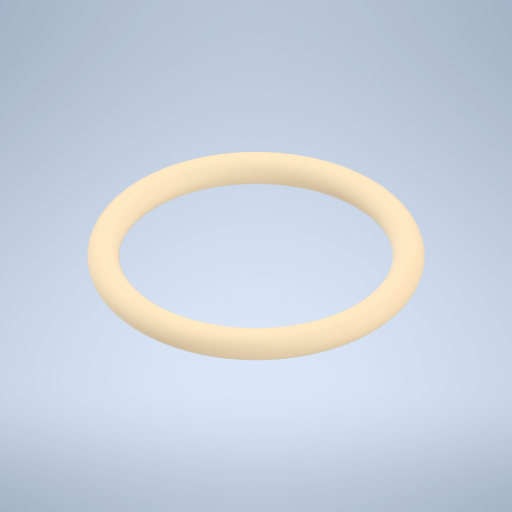
# Autodesk Inventor part: dummy_ling_string
Saved by Autodesk Inventor 2024.3 (Build 283343000, 343)
## iProperties
Created: 2024-09-12
Part Number: dummy_ling_string
Material: Generic
Document SubType Name: Modeling
Designer: gihyeok2
Density: 1 g/cm^3
Appearance: Default
Author: gihyeok2
Autodesk Inventor part; units mm, degrees
ref_plane "YZ Plane" through (0, 0, 0) normal (1, 0, 0) x (0, 1, 0)
ref_plane "XZ Plane" through (0, 0, 0) normal (0, 1, 0) x (-1, 0, 0)
ref_plane "XY Plane" through (0, 0, 0) normal (0, 0, 1) x (1, 0, 0)
sketch "Sketch3" plane through (0, 0, 0) normal (1, 0, 0) x (0, 1, 0)
  circle A0 centre (0, -2.35) radius 0.25
  line L0 (0, -2.35) -> (0, 0) construction
  line L1 (0, 0) -> (6.6454, 0) construction
  dimension "d3" = 0.5
  dimension "d4" = 2.35
  constraints: 4 end point, 1 centre point, 1 horizontal, 1 vertical
  measures "d3" diameter of A0
  measures "d4" distance of L0.start L0.end
revolve "Revolution1" add sketch "Sketch3" angle 360 about axis through (0, 0, 0) along (0, 1, 0)
body "Solid1"
